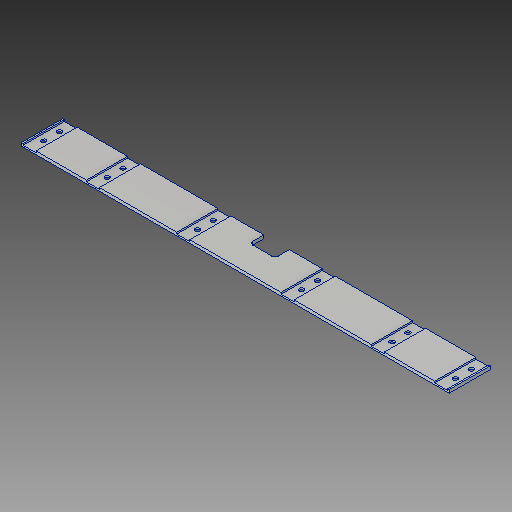
# Autodesk Inventor part: 앞뒷판_중간
Saved by Autodesk Inventor 2017 (Build 210142000, 142)
## iProperties
Part Number: 앞뒷판_중간
Material: 알루미늄 6061
Document SubType Name: Modeling
Designer: minom
Density: 2.7 g/cm^3
Appearance: 알루미늄 - 평지
Mass: 33.4568 g
Surface Area: 151.291 cm^2
Volume: 12.3914 cm^3
Author: minom
Autodesk Inventor part; units mm, degrees
ref_plane "YZ Plane" through (0, 0, 0) normal (1, 0, 0) x (0, 1, 0)
ref_plane "XZ Plane" through (0, 0, 0) normal (0, 1, 0) x (-1, 0, 0)
ref_plane "XY Plane" through (0, 0, 0) normal (0, 0, 1) x (1, 0, 0)
sketch "스케치1" plane through (0, 0, 0) normal (0, 1, 0) x (-1, 0, 0)
  line L0 (0, 0) -> (-270, 0)
  line L1 (-270, 0) -> (-270, -26)
  line L2 (-270, -26) -> (0, -26)
  line L3 (0, -26) -> (0, 0)
  dimension "d0" = 270
  dimension "d1" = 26
  constraints: 8 end point, 2 parallel, 1 horizontal, 1 perpendicular
  measures "d0" distance of L2.end L1.end
  measures "d1" distance of L1.end L0.end
extrude "돌출1" add sketch "스케치1" along normal blind 2
sketch "스케치2" plane through (0, 2, 0) normal (0, 1, 0) x (1, 0, 0)
  line L0 (0, 0) -> (270, 0) projected
  line L1 (270, 0) -> (270, 26) projected
  line L2 (270, 26) -> (0, 26) projected
  line L3 (0, 26) -> (0, 0) projected
  line L4 (1, 26) -> (1, 0)
  line L5 (9.2, 26) -> (9.2, 0)
  line L6 (269, 26) -> (269, 0)
  line L7 (260.8, 26) -> (260.8, 0)
  line L8 (0, 0) -> (270, 0) projected
  line L9 (270, 26) -> (0, 26) projected
  line L10 (260.8, 0) -> (269, 0)
  line L11 (260.8, 26) -> (269, 26)
  line L12 (0, 0) -> (40, 0)
  line L13 (40, 0) -> (41, 0)
  line L14 (41, 0) -> (41, 26)
  line L15 (41, 0) -> (49.2, 0)
  line L16 (49.2, 0) -> (49.2, 26)
  line L17 (270, 0) -> (270, 0)
  line L18 (270, 0) -> (229, 0)
  line L19 (229, 0) -> (220.8, 0)
  line L20 (220.8, 0) -> (220.8, 26)
  line L21 (229, 0) -> (229, 26)
  line L22 (229, 26) -> (220.8, 26)
  line L23 (41, 26) -> (49.2, 26)
  line L24 (9.2, 0) -> (1, 0)
  line L25 (9.2, 26) -> (1, 26)
  line L26 (1, 0) -> (1, 26)
  dimension "d19" = 8.2
  dimension "d20" = 1
  dimension "d21" = 8.2
  dimension "d22" = 40
  dimension "d23" = 1
  dimension "d24" = 8.2
  dimension "d26" = 8.2
  dimension "d29" = 41
  constraints: 42 end point, 4 perpendicular, 4 vertical, 3 collinear, 3 point on line, 2 horizontal, 1 parallel, 17 other
  measures "d19" distance between parallel lines of L5 L4
  measures "d20" distance between parallel lines of L1 L6
  measures "d21" distance between parallel lines of L6 L7
  measures "d22" distance of L12.start L12.end
  measures "d23" distance of L12.end L13.end
  measures "d24" distance of L13.end L15.end
  measures "d26" distance of L18.end L19.end
  measures "d29" distance between parallel lines of L1 L21
extrude "돌출3" cut sketch "스케치2" against normal blind 1 contours L4 L2 L5 L0 | L14 L2 L16 L0 | L20 L2 L21 L0 | L7 L2 L6 L0
sketch "스케치5" plane through (0, 0, 0) normal (0, -1, 0) x (1, 0, 0)
  line L0 (0, 0) -> (270, 0) projected
  line L1 (0, -26) -> (0, 0) projected
  line L2 (270, -26) -> (0, -26) projected
  line L3 (270, 0) -> (270, -26) projected
  line L4 (0, 0) -> (270, 0) projected
  line L5 (270, -26) -> (0, -26) projected
  line L6 (127, -26) -> (127, -19)
  line L7 (129, -17) -> (141, -17)
  line L8 (143, -19) -> (143, -26)
  arc A0 (129, -17) -> (127, -19) centre (129, -19) ccw
  arc A1 (143, -19) -> (141, -17) centre (141, -19) ccw
  point P0 (127, -17)
  point P1 (143, -17)
  dimension "d39" = 9
  dimension "d40" = 16
  dimension "d70" = 127
  dimension "d71" = 2
  dimension "d72" = 2
  constraints: 6 end point, 6 point on line, 4 point on circle, 4 tangent, 2 centre point, 2 perpendicular, 1 vertical
  measures "d39" distance between parallel lines of L5 L7
  measures "d40" distance between parallel lines of L6 L8
  measures "d70" distance between parallel lines of L6 L1
  measures "d71" radius of A0
  measures "d72" radius of A1
sketch "스케치6" plane through (0, 0, 0) normal (0, -1, 0) x (1, 0, 0)
  line L0 (1, -26) -> (9.2, -26) projected
  line L1 (1, 0) -> (1, -26) projected
  line L2 (9.2, 0) -> (1, 0) projected
  line L3 (9.2, -26) -> (9.2, 0) projected
  line L4 (49.2, 0) -> (41, 0) projected
  line L5 (49.2, -26) -> (49.2, 0) projected
  line L6 (41, -26) -> (49.2, -26) projected
  line L7 (41, 0) -> (41, -26) projected
  line L8 (220.8, -26) -> (229, -26) projected
  line L9 (220.8, 0) -> (220.8, -26) projected
  line L10 (229, 0) -> (220.8, 0) projected
  line L11 (229, -26) -> (229, 0) projected
  line L12 (269, -26) -> (269, 0) projected
  line L13 (260.8, -26) -> (269, -26) projected
  line L14 (260.8, 0) -> (260.8, -26) projected
  line L15 (269, 0) -> (260.8, 0) projected
  circle A0 centre (5.1, -9) radius 1.5
  circle A1 centre (5.1, -19) radius 1.5
  circle A2 centre (45.1, -9) radius 1.5
  circle A3 centre (45.1, -19) radius 1.5
  circle A4 centre (224.9, -9) radius 1.5
  circle A5 centre (224.9, -19) radius 1.5
  circle A6 centre (264.9, -19) radius 1.5
  circle A7 centre (264.9, -9) radius 1.5
  point P0 (0, 0)
  dimension "d43" = 3
  dimension "d44" = 3
  dimension "d45" = 3
  dimension "d46" = 3
  dimension "d47" = 3
  dimension "d48" = 3
  dimension "d49" = 3
  dimension "d50" = 3
  dimension "d51" = 4.1
  dimension "d52" = 4.1
  dimension "d53" = 4.1
  dimension "d54" = 4.1
  dimension "d55" = 4.1
  dimension "d56" = 4.1
  dimension "d57" = 4.1
  dimension "d58" = 4.1
  dimension "d59" = 9
  dimension "d60" = 7
  dimension "d61" = 7
  dimension "d62" = 9
  dimension "d63" = 9
  dimension "d64" = 7
  dimension "d65" = 7
  dimension "d66" = 9
  constraints: 8 centre point
  measures "d43" diameter of A0
  measures "d44" diameter of A1
  measures "d45" diameter of A2
  measures "d46" diameter of A3
  measures "d47" diameter of A4
  measures "d48" diameter of A5
  measures "d49" diameter of A6
  measures "d50" diameter of A7
  measures "d51" distance from line of L1 A0.centre
  measures "d52" distance from line of L3 A1.centre
  measures "d53" distance from line of L7 A2.centre
  measures "d54" distance from line of L5 A3.centre
  measures "d55" distance from line of L9 A4.centre
  measures "d56" distance from line of L11 A5.centre
  measures "d57" distance from line of L14 A6.centre
  measures "d58" distance from line of L12 A7.centre
  measures "d59" distance from line of L15 A7.centre
  measures "d60" distance from line of L13 A6.centre
  measures "d61" distance from line of L8 A5.centre
  measures "d62" distance from line of L10 A4.centre
  measures "d63" distance from line of L4 A2.centre
  measures "d64" distance from line of L6 A3.centre
  measures "d65" distance from line of L0 A1.centre
  measures "d66" distance from line of L2 A0.centre
extrude "돌출6" cut sketch "스케치6" against normal blind 10 contours A0 | A1 | A2 | A3 | A4 | A5 | A6 | A7
extrude "돌출7" cut sketch "스케치5" against normal blind 2 contours L6 A0 L7 A1 L8 L2
sketch "스케치7" plane through (0, 2, 0) normal (0, 1, 0) x (1, 0, 0)
  line L0 (127, 19) -> (127, 26) projected
  line L1 (127, 26) -> (49.2, 26) projected
  line L2 (49.2, 26) -> (49.2, 0) projected
  line L3 (49.2, 0) -> (220.8, 0) projected
  line L4 (220.8, 0) -> (220.8, 26) projected
  line L5 (220.8, 26) -> (143, 26) projected
  line L6 (143, 26) -> (143, 19) projected
  arc A0 (141, 17) -> (143, 19) centre (141, 19) ccw projected
  line L7 (141, 17) -> (129, 17) projected
  arc A1 (127, 19) -> (129, 17) centre (129, 19) ccw projected
  line L8 (49.2, 0) -> (220.8, 0) projected
  line L9 (270, 26) -> (143, 26) projected
  line L10 (172, 0) -> (163.8, 0)
  line L11 (163.8, 0) -> (163.8, 26)
  line L12 (163.8, 26) -> (172, 26)
  line L13 (172, 26) -> (172, 0)
  line L14 (127, 26) -> (49.2, 26) projected
  line L15 (106.2, 0) -> (98, 0)
  line L16 (98, 0) -> (98, 26)
  line L17 (98, 26) -> (106.2, 26)
  line L18 (106.2, 26) -> (106.2, 0)
  line L19 (270, 0) -> (270, 26) projected
  line L20 (0, 26) -> (0, 0) projected
  dimension "d75" = 8.2
  dimension "d76" = 8.2
  dimension "d77" = 98
  dimension "d78" = 98
  constraints: 16 end point, 4 parallel, 4 point on line, 2 horizontal, 2 perpendicular
  measures "d75" distance of L11.end L12.end
  measures "d76" distance of L16.end L17.end
  measures "d77" distance between parallel lines of L13 L19
  measures "d78" distance between parallel lines of L16 L20
extrude "돌출8" cut sketch "스케치7" against normal blind 1 contours L18 L3 L16 L1 | L11 L5 L13 L3
sketch "스케치8" plane through (0, 1, 0) normal (0, 1, 0) x (1, 0, 0)
  circle A0 centre (167.9, 19) radius 1.5
  circle A1 centre (167.9, 9) radius 1.5
  circle A2 centre (102.1, 9) radius 1.5
  circle A3 centre (102.1, 19) radius 1.5
  line L0 (163.8, 26) -> (172, 26) projected
  line L1 (172, 26) -> (172, 0) projected
  line L2 (163.8, 0) -> (163.8, 26) projected
  line L3 (106.2, 26) -> (106.2, 0) projected
  line L4 (98, 0) -> (98, 26) projected
  line L5 (98, 26) -> (106.2, 26) projected
  point P0 (0, 0)
  dimension "d81" = 3
  dimension "d82" = 3
  dimension "d83" = 3
  dimension "d84" = 3
  dimension "d85" = 7
  dimension "d86" = 4.1
  dimension "d87" = 4.1
  dimension "d88" = 10
  dimension "d89" = 4.1
  dimension "d90" = 4.1
  dimension "d91" = 7
  dimension "d92" = 10
  constraints: 4 centre point
  measures "d81" diameter of A0
  measures "d82" diameter of A1
  measures "d83" diameter of A2
  measures "d84" diameter of A3
  measures "d85" distance from line of L0 A0.centre
  measures "d86" distance from line of L1 A0.centre
  measures "d87" distance from line of L2 A1.centre
  measures "d88" distance of A0.centre A1.centre
  measures "d89" distance from line of L3 A3.centre
  measures "d90" distance from line of L4 A2.centre
  measures "d91" distance from line of L5 A3.centre
  measures "d92" distance of A2.centre A3.centre
extrude "돌출9" cut sketch "스케치8" against normal blind 1
